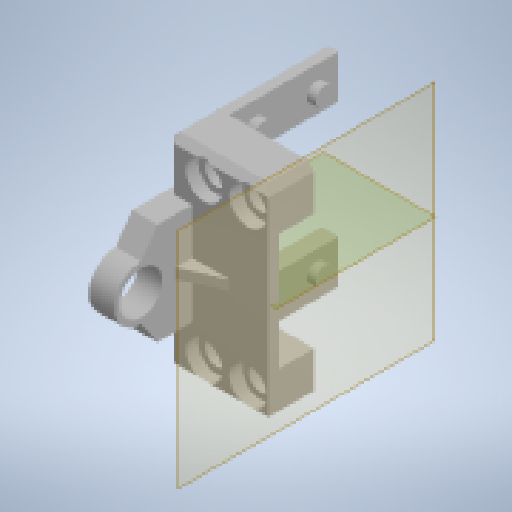
# Autodesk Inventor part: Sensor_Adapter_v2
Saved by Autodesk Inventor 2023 (Build 270158000, 158)
## iProperties
Created: 2022-09-16
Part Number: Sensor_Adapter_v2
Material: Generic
Document SubType Name: Modeling
Designer: think
Density: 1 g/cm^3
Appearance: Default
Author: think
Autodesk Inventor part; units mm, degrees
ref_plane "YZ Plane" through (0, 0, 0) normal (1, 0, 0) x (0, 1, 0)
ref_plane "XZ Plane" through (0, 0, 0) normal (0, 1, 0) x (-1, 0, 0)
ref_plane "Work Plane2" through (-30, 13, 10.5) normal (0, 0, 1) x (1, 0, 0)
sketch "Sketch1" plane through (0, 0, 0) normal (0, 0, 1) x (1, 0, 0)
  line L0 (0, 13) -> (-30, 13) projected
  line L1 (0, 0) -> (-30, 0)
  line L2 (-30, 0) -> (-30, 12.75)
  line L3 (-30, 12.75) -> (0, 12.75)
  line L4 (0, 12.75) -> (0, 0)
  circle A0 centre (-19, 7) radius 5.4 projected
  circle A1 centre (-6, 7) radius 5.4 projected
  circle A2 centre (-19, 7) radius 5.9
  circle A3 centre (-6, 7) radius 5.9
  point P0 (-4.6781, 12.75)
  point P1 (-7.3219, 12.75)
  point P2 (-17.6781, 12.75)
  point P3 (-20.3219, 12.75)
  dimension "d0" = 0.25
  dimension "d1" = 0.5
  constraints: 8 end point, 2 centre point, 2 coincident, 2 parallel, 1 equal radius, 1 horizontal, 1 perpendicular, 1 vertical alignment
  measures "d0" distance between parallel lines of L0 L3
  measures "d1" radial gap between concentric circles of A2 A0
extrude "Extrusion1" add sketch "Sketch1" along normal up to surface (10.5 mm away) contours L1 L2 L3 A2 A3 L4 | A3 L3 | L3 A3 | A2 L3 | L3 A2 | A0 | A1
sketch "Sketch2" plane through (-30, 0, 0) normal (-1, 0, 0) x (0, 0, 1)
  line L0 (0, 0) -> (10.5, 0) projected
  line L1 (0, 0) -> (-32.2, 0)
  line L2 (-32.2, 0) -> (-32.2, 12.75)
  line L3 (-32.2, 12.75) -> (0, 12.75)
  line L4 (0, 12.75) -> (0, 0)
  line L5 (0, 12.75) -> (10.5, 12.75) projected
  line L6 (-32.5, 60) -> (-32.5, 0) projected
  point P0 (10, 0)
  point P1 (10, 12.75)
  dimension "d4" = 0.3
  constraints: 8 end point, 2 parallel, 1 horizontal, 1 perpendicular, 1 point on line
  measures "d4" distance between parallel lines of L6 L2
extrude "Extrusion2" add sketch "Sketch2" against normal blind 5
sketch "Sketch3" plane through (-25, 0, 0) normal (1, 0, 0) x (0, 0, -1)
  circle A0 centre (7.75, 7) radius 2.8
  circle A1 centre (25.75, 7) radius 2.8
  circle A2 centre (7.5, 7) radius 3.3 projected
  circle A3 centre (25.5, 7) radius 3.3 projected
  point P0 (0, 0)
  dimension "d46" = 0.25
  dimension "d47" = 0.25
  dimension "d48" = 5.6
  constraints: 2 centre point, 2 horizontal alignment, 1 equal radius
  measures "d46" distance of A3.centre A1.centre
  measures "d47" distance of A0.centre A2.centre
  measures "d48" diameter of A0
extrude "Extrusion3" add sketch "Sketch3" along normal blind 2.5 contours A0 | A1
ref_plane "Work Plane1" through (-30, 30, 10.5) normal (0, -1, 0) x (1, 0, 0)
mirror "Mirror1" about plane through (-30, 30, 10.5) normal (0, -1, 0) of "Extrusion1", "Extrusion2", "Extrusion3"
sketch "Sketch5" plane through (-30, 60, 10.5) normal (0, 0, 1) x (1, 0, 0)
  line L0 (30, 0) -> (0, 0) projected
  line L1 (30, -60) -> (0, -60) projected
  line L2 (0, 0) -> (0, -60)
  line L3 (30, -60) -> (30, -47.25) projected
  line L4 (30, -60) -> (30, 0)
  constraints: 4 end point, 1 collinear, 1 vertical
extrude "Extrusion4" add sketch "Sketch5" along normal blind 3
ref_plane "Work Plane3" through (0, 30, 13.5) normal (1, 0, 0) x (0, 0, -1)
sketch "Sketch6" plane through (-30, 30, 13.5) normal (1, 0, 0) x (0, 0, -1)
  line L0 (0, 30) -> (-15, 8)
  line L1 (-15, -8) -> (0, -30)
  line L2 (-15, 8) -> (-15, -8)
  circle A0 centre (-15, 0) radius 8
  circle A1 centre (-15, 0) radius 6.25
  line L3 (0, 30) -> (0, -30)
  line L4 (-10.2273, -15) -> (0, -15)
  line L5 (-10.2273, 15) -> (0, 15)
  line L6 (0, -30) -> (0, 30) projected
  point P0 (13.5, -30)
  point P1 (-15, 0)
  point P2 (0, 0)
  point P3 (-5.1136, 15)
  point P4 (-5.1136, -15)
  point P5 (0, 15)
  point P6 (-15, -8)
  point P7 (-15, -6.25)
  point P8 (-15, 6.25)
  dimension "d13" = 16
  dimension "d15" = 12.5
  dimension "d41" = 15
  dimension "d42" = 30
  constraints: 12 end point, 4 midpoint, 4 point on line, 2 coincident, 1 centre point, 1 equal length, 1 horizontal, 1 parallel, 1 vertical, 1 vertical alignment, 3 other
  measures "d13" distance of L1.start L0.end
  measures "d15" diameter of A1
  measures "d41" distance of point (0, 0) point (-15, 0)
  measures "d42" distance of point (-5.114, 15) point (-5.114, -15)
extrude "Extrusion5" add sketch "Sketch6" along normal blind 7.5 contours L5 L3 L4 L1 A0 L0 | A0 L2 A1 | L2 A1 A0
sketch "Sketch7" plane through (-30, 60, 13.5) normal (0, 0, 1) x (1, 0, 0)
  circle A0 centre (24, -7) radius 5.4 projected
  circle A1 centre (11, -7) radius 5.4 projected
  circle A2 centre (24, -53) radius 5.4 projected
  circle A3 centre (11, -53) radius 5.4 projected
  circle A4 centre (24, -7) radius 6.9
  circle A5 centre (24, -53) radius 6.9
  circle A6 centre (11, -7) radius 6.9
  circle A7 centre (11, -53) radius 6.9
  point P0 (30, -60)
  dimension "d21" = 1.5
  constraints: 4 centre point, 3 equal radius, 2 coincident, 2 concentric
  measures "d21" radial gap between concentric circles of A2 A5
extrude "Extrusion6" cut sketch "Sketch7" along normal blind 25.25 and the other way blind 3.75 contours A0 | A1 | A2 | A3
chamfer "Chamfer2" distance 2 angle 45 8 edges at (-15, 60, 13.5) (-30, 52.5, 13.5) (-30, 7.5, 13.5) (-15, 0, 13.5) (-30, 60, -9.35) (-30, 0, -9.35) (0, 60, 6.75) (0, 0, 6.75)
sketch "Sketch10" plane through (-19, 7, 9.75) normal (0, 0, 1) x (1, 0, 0)
  circle A0 centre (0, 0) radius 2.5 projected
  circle A1 centre (13, 0) radius 2.5 projected
  circle A2 centre (0, 46) radius 2.5 projected
  circle A3 centre (13, 46) radius 2.5 projected
  circle A4 centre (0, 46) radius 3.5
  circle A5 centre (13, 46) radius 3.5
  circle A6 centre (0, 0) radius 3.5
  circle A7 centre (13, 0) radius 3.5
  point P0 (19, -7)
  dimension "d38" = 7
  constraints: 4 centre point, 4 coincident, 3 equal radius
  measures "d38" diameter of A5
extrude "Extrusion9" cut sketch "Sketch10" against normal blind 28 contours A0 | A1 | A2 | A3 | A4 | A5 | A6 | A7
sketch "Sketch12" plane through (-30, 30, 10.5) normal (0, -1, 0) x (1, 0, 0)
  line L0 (7.5, 18) -> (7.5, 13.2273) projected
  line L1 (7.5, 18) -> (7.5, 18) projected
  line L2 (7.5, 13.2273) -> (7.5, 18) projected
  line L3 (7.5, 3) -> (7.5, 13.2273) projected
  line L4 (7.5, 13.2273) -> (7.5, 3) projected
  line L5 (7.5, 24.25) -> (7.5, 11.75) projected
  line L6 (26.0396, 3) -> (21.9604, 3) projected
  line L7 (13.0396, 3) -> (8.9604, 3) projected
  line L8 (8.9604, 3) -> (13.0396, 3) projected
  line L9 (21.9604, 3) -> (26.0396, 3) projected
  line L10 (7.5, 8) -> (18.6, 3)
  line L11 (30, 3) -> (26.0396, 3) projected
  line L12 (26.0396, 3) -> (30, 3) projected
  line L13 (13.0396, 3) -> (21.9604, 3) projected
  line L14 (2, 3) -> (8.9604, 3) projected
  line L15 (2, 3) -> (7.5, 3) projected
  line L16 (7.5, 3) -> (2, 3) projected
  line L17 (8.9604, 3) -> (2, 3) projected
  line L18 (21.9604, 3) -> (13.0396, 3) projected
  point P0 (30, -10.5)
  point P1 (29.4, 3)
  point P2 (18.6, 3)
  point P3 (29.4, 3)
  point P4 (5.6, 3)
  point P5 (16.4, 3)
  point P6 (16.4, 3)
  point P7 (18.6, 3)
  point P8 (7.5, 8)
  point P9 (22.5, 3)
  dimension "d43" = 5
  constraints: 2 end point, 1 coincident, 1 point on line
  measures "d43" vertical distance of point (29.4, 3) L10.start
extrude "Extrusion10" add sketch "Sketch12" along normal mid plane 3
body "Solid1"
